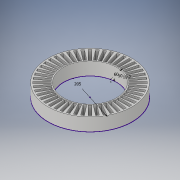
# Autodesk Inventor part: ring as whole
Saved by Autodesk Inventor 2018 (Build 220112000, 112)
## iProperties
Created: 2024-05-06
Part Number: ring as whole
Material: Generic
Document SubType Name: Modeling
Designer: neo
Density: 1 g/cm^3
Appearance: Default
Author: neo
Autodesk Inventor part; units mm, degrees
ref_plane "YZ Plane" through (0, 0, 0) normal (1, 0, 0) x (0, 1, 0)
ref_plane "XZ Plane" through (0, 0, 0) normal (0, 1, 0) x (-1, 0, 0)
ref_plane "XY Plane" through (0, 0, 0) normal (0, 0, 1) x (1, 0, 0)
sketch "Sketch1" plane through (0, 0, 0) normal (0, 1, 0) x (-1, 0, 0)
  circle A0 centre (0, 0) radius 102.5
  circle A1 centre (0, 0) radius 162.5
  line L0 (0, -102.5) -> (0, -162.5)
  line L1 (5.1, -106.5) -> (-5.1, -106.5)
  line L2 (-5.1, -106.5) -> (-5.1, -156.5)
  line L3 (-5.1, -156.5) -> (5.1, -156.5)
  line L4 (5.1, -156.5) -> (5.1, -106.5)
  dimension "d0" = 60
  dimension "d1" = 205
  dimension "d3" = 10.2
  dimension "d4" = 50
  dimension "d5" = 4
  constraints: 10 end point, 2 coincident, 2 parallel, 2 vertical alignment, 1 horizontal, 1 perpendicular, 1 vertical, 5 other
  measures "d3" distance between parallel lines of L2 L4
  measures "d4" distance of L3.end L1.start
  measures "d5" distance from line of L1 L0.start
extrude "Extrusion1" add sketch "Sketch1" along normal blind 50 contours A1 | L1 L4 L3 L0 | L0 L3 L2 L1
extrude "Extrusion2" cut sketch "Sketch1" along normal blind 50 contours L1 L4 L3 L0 | L0 L3 L2 L1
pattern_circular "Circular Pattern1" count 48 over 360 about axis through (0, 0, 0) along (0, 1, 0) of "Extrusion2"
body "Solid1"
